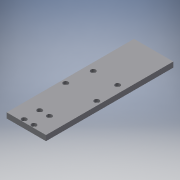
# Autodesk Inventor part: suporte_cabeça_superior
Saved by Autodesk Inventor 2018 (Build 220112000, 112)
## iProperties
Created: 2018-05-17
Part Number: suporte_cabeça_superior
Material: Genérico
Document SubType Name: Modeling
Designer: Usuario
Density: 1 g/cm^3
Appearance: Padrão
Author: Usuario
Autodesk Inventor part; units mm, degrees
ref_plane "YZ Plane" through (0, 0, 0) normal (1, 0, 0) x (0, 1, 0)
ref_plane "XZ Plane" through (0, 0, 0) normal (0, 1, 0) x (-1, 0, 0)
ref_plane "XY Plane" through (0, 0, 0) normal (0, 0, 1) x (1, 0, 0)
sketch "Esboço2" plane through (0, 0, 0) normal (0, 0, 1) x (1, 0, 0)
  circle A0 centre (11.015, 104.9) radius 1.621 construction
  line L0 (17.015, 98.9) -> (17.015, 110.9) construction
  line L1 (17.015, 110.9) -> (5.015, 110.9) construction
  line L2 (5.015, 110.9) -> (5.015, 98.9) construction
  line L3 (5.015, 98.9) -> (17.015, 98.9) construction
  circle A1 centre (54.985, 104.9) radius 1.621 construction
  line L4 (48.985, 110.9) -> (48.985, 98.9) construction
  line L5 (48.985, 98.9) -> (60.985, 98.9) construction
  line L6 (60.985, 98.9) -> (60.985, 110.9) construction
  line L7 (60.985, 110.9) -> (48.985, 110.9) construction
  circle A2 centre (5, 61.2) radius 1.621 construction
  line L8 (-1, 67.2) -> (-1, 55.2) construction
  line L9 (-1, 55.2) -> (11, 55.2) construction
  line L10 (11, 55.2) -> (11, 67.2) construction
  line L11 (11, 67.2) -> (-1, 67.2) construction
  circle A3 centre (61, 61.2) radius 1.621 construction
  line L12 (67, 55.2) -> (67, 67.2) construction
  line L13 (67, 67.2) -> (55, 67.2) construction
  line L14 (55, 67.2) -> (55, 55.2) construction
  line L15 (55, 55.2) -> (67, 55.2) construction
  circle A4 centre (41.8302, -33) radius 1.621 construction
  circle A5 centre (24.1698, -5) radius 1.621 construction
  circle A6 centre (24.1698, -33) radius 1.621 construction
  circle A7 centre (41.8302, -5) radius 1.621 construction
  line L16 (46.8302, 0) -> (46.8302, -38) construction
  line L17 (19.1698, 0) -> (46.8302, 0) construction
  line L18 (19.1698, -38) -> (19.1698, 0) construction
  line L19 (19.1698, -38) -> (46.8302, -38) construction
  line L20 (-1.4393, 191.951) -> (-2.5, 191.951) construction
  line L21 (-2.5, 191.951) -> (-2.5, 190.8903) construction
  line L22 (67.4393, -37.951) -> (68.5, -37.951) construction
  line L23 (68.5, -37.951) -> (68.5, -36.8903) construction
  line L24 (-2.5, 191.951) -> (68.5, 191.951)
  line L25 (68.5, 191.951) -> (68.5, -37.951)
  line L26 (68.5, -37.951) -> (-2.5, -37.951)
  line L27 (-2.5, -37.951) -> (-2.5, 191.951)
  point P0 (0, 0)
  dimension "d12" = 71
  constraints: 16 end point, 3 horizontal, 3 perpendicular, 2 parallel
  measures "d12" distance of L20.end L24.end
extrude "Extrusão2" add sketch "Esboço2" along normal blind 9.5
sketch "Esboço3" plane through (0, 0, 9.5) normal (0, 0, 1) x (1, 0, 0)
  circle A0 centre (41.8302, -5) radius 1.621 construction
  circle A1 centre (24.1698, -5) radius 1.621 construction
  circle A2 centre (41.8302, -33) radius 1.621 construction
  circle A3 centre (24.1698, -33) radius 1.621 construction
  circle A4 centre (54.985, 104.9) radius 1.621 construction
  circle A5 centre (11.015, 104.9) radius 1.621 construction
  circle A6 centre (5, 61.2) radius 1.621 construction
  circle A7 centre (61, 61.2) radius 1.621 construction
  point P0 (0, 0)
hole "Furo1" at (11.015, 104.9, 9.5) at (54.985, 104.9, 9.5) at (5, 61.2, 9.5) at (61, 61.2, 9.5) at (24.1698, -5, 9.5) at (41.8302, -5, 9.5) at (24.1698, -33, 9.5) at (41.8302, -33, 9.5) direction (0, 0, -1) diameter 4 end through all counterbore diameter 9 counterbore depth 5.5
